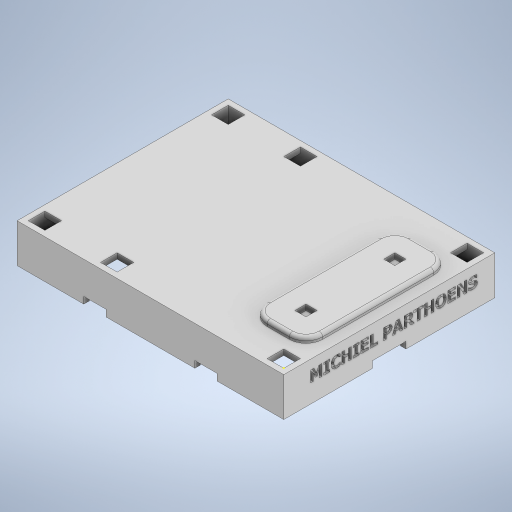
# Autodesk Inventor part: bovenkant
Saved by Autodesk Inventor 2023 (Build 270158000, 158)
## iProperties
Created: 2023-06-01
Part Number: bovenkant
Material: Generic
Document SubType Name: Modeling
Designer: Prestige
Density: 1 g/cm^3
Appearance: Default
Author: Prestige
Autodesk Inventor part; units mm, degrees
ref_plane "YZ Plane" through (0, 0, 0) normal (1, 0, 0) x (0, 1, 0)
ref_plane "XZ Plane" through (0, 0, 0) normal (0, 1, 0) x (-1, 0, 0)
ref_plane "XY Plane" through (0, 0, 0) normal (0, 0, 1) x (1, 0, 0)
sketch "Sketch1" plane through (0, 0, 0) normal (0, 1, 0) x (-1, 0, 0)
  line L0 (0, 0) -> (230, 0)
  line L1 (230, 0) -> (230, -180)
  line L2 (230, -180) -> (0, -180)
  line L3 (0, -180) -> (0, 0)
  line L4 (235, -185) -> (-5, -185)
  line L5 (-5, -185) -> (-5, 5)
  line L6 (-5, 5) -> (235, 5)
  line L7 (235, 5) -> (235, -185)
  line L8 (235, -75) -> (230, -75)
  line L9 (230, -75) -> (230, -105)
  line L10 (230, -105) -> (235, -105)
  line L11 (235, -105) -> (235, -75)
  line L12 (175, -180) -> (155, -180)
  line L13 (155, -180) -> (155, -185)
  line L14 (155, -185) -> (175, -185)
  line L15 (175, -185) -> (175, -180)
  line L16 (115, -180) -> (95, -180)
  line L17 (95, -185) -> (115, -185)
  line L18 (-5, -73.4747) -> (0, -73.4747)
  line L19 (0, -73.4747) -> (0, -111.2886)
  line L20 (0, -111.2886) -> (-5, -111.2886)
  line L21 (-5, -111.2886) -> (-5, -73.4747)
  line L22 (175, 0) -> (155, 0)
  line L23 (155, 0) -> (155, 5)
  line L24 (155, 5) -> (175, 5)
  line L25 (175, 5) -> (175, 0)
  line L26 (75, 0) -> (55, 0)
  line L27 (55, 0) -> (55, 5)
  line L28 (55, 5) -> (75, 5)
  line L29 (75, 5) -> (75, 0)
  line L30 (75, -180) -> (55, -180)
  line L31 (55, -180) -> (55, -185)
  line L32 (55, -185) -> (75, -185)
  line L33 (75, -185) -> (75, -180)
  point P0 (232.5, -75)
  point P1 (232.5, -105)
  point P2 (175, 2.5)
  point P3 (155, 2.5)
  point P4 (55, 2.5)
  point P5 (75, 2.5)
  point P6 (155, -182.5)
  point P7 (175, -182.5)
  point P8 (55, -182.5)
  point P9 (75, -182.5)
  point P10 (-5, -111.2886)
  point P11 (0, -73.4747)
  dimension "d0" = 180
  dimension "d1" = 230
  dimension "d2" = 5
  dimension "d3" = 5
  dimension "d4" = 5
  dimension "d5" = 5
  dimension "d6" = 30
  dimension "d7" = 75
  dimension "d8" = 75
  dimension "d9" = 20
  dimension "d10" = 20
  dimension "d12" = 20
  dimension "d14" = 80
  dimension "d15" = 55
  dimension "d16" = 55
  dimension "d17" = 20
  dimension "d18" = 80
  constraints: 68 end point, 17 parallel, 13 point on line, 11 midpoint, 9 horizontal, 8 perpendicular
  measures "d0" distance of L2.end L0.start
  measures "d1" distance of L0.start L0.end
  measures "d2" distance between parallel lines of L1 L7
  measures "d3" distance between parallel lines of L2 L4
  measures "d4" distance between parallel lines of L3 L5
  measures "d5" distance between parallel lines of L0 L6
  measures "d6" distance from line of point (232.5, -75) L10
  measures "d7" distance between parallel lines of L0 L8
  measures "d8" distance from line of L2 point (232.5, -105)
  measures "d9" distance of point (175, 2.5) point (155, 2.5)
  measures "d10" distance of point (55, 2.5) point (75, 2.5)
  measures "d12" distance of point (155, -182.5) point (175, -182.5)
  measures "d14" distance between parallel lines of L23 L29
  measures "d15" distance between parallel lines of L1 L25
  measures "d16" distance between parallel lines of L1 L15
  measures "d17" distance of point (55, -182.5) point (75, -182.5)
  measures "d18" distance from line of point (155, -182.5) L33
extrude "Extrusion1" add sketch "Sketch1" along normal blind 6 contours L3 L18 L5 L6 L27 L0 | L29 L6 L23 L0 | L3 L2 L31 L4 L5 L20 | L25 L6 L7 L8 L1 L0 | L2 L13 L4 L33 | L10 L7 L4 L15 L2 L1
sketch "Sketch2" plane through (0, 6, 0) normal (0, 1, 0) x (1, 0, 0)
  line L0 (0, 180) -> (0, 111.2886) projected
  line L1 (-175, 0) -> (-230, 0) projected
  line L2 (0, 180) -> (-230, 180)
  line L3 (-230, 180) -> (-230, 0)
  line L4 (-230, 0) -> (0, 0)
  line L5 (0, 0) -> (0, 180)
  line L6 (-235, 75) -> (-235, -5) projected
  line L7 (5, 111.2886) -> (5, 185) projected
  line L8 (-235, -5) -> (5, -5)
  line L9 (5, -5) -> (5, 185)
  line L10 (5, 185) -> (-235, 185)
  line L11 (-235, 185) -> (-235, -5)
  point P0 (0, 0)
  constraints: 16 end point, 4 parallel, 2 horizontal, 2 perpendicular
extrude "Extrusion2" add sketch "Sketch2" along normal blind 24
sketch "Sketch3" plane through (0, 30, 0) normal (0, 1, 0) x (1, 0, 0)
  line L0 (-235, -5) -> (5, -5) projected
  line L1 (5, 185) -> (-235, 185) projected
  line L2 (-235, -5) -> (5, -5)
  line L3 (5, -5) -> (5, 185)
  line L4 (5, 185) -> (-235, 185)
  line L5 (-235, 185) -> (-235, -5)
  point P0 (0, 0)
  constraints: 8 end point, 2 parallel, 1 horizontal, 1 perpendicular
extrude "Extrusion3" add sketch "Sketch3" along normal blind 5
sketch "Sketch4" plane through (0, 35, 0) normal (0, 1, 0) x (1, 0, 0)
  line L0 (-5, 25) -> (-55, 25)
  line L1 (-55, 25) -> (-55, 155)
  line L2 (-55, 155) -> (-5, 155)
  line L3 (-5, 155) -> (-5, 25)
  line L4 (5, 185) -> (-235, 185) projected
  line L5 (-235, -5) -> (5, -5) projected
  line L6 (5, -5) -> (5, 185) projected
  point P0 (0, 0)
  dimension "d25" = 130
  dimension "d26" = 30
  dimension "d27" = 30
  dimension "d28" = 10
  dimension "d29" = 50
  constraints: 8 end point, 2 parallel, 1 horizontal, 1 perpendicular
  measures "d25" distance of L0.end L1.end
  measures "d26" distance between parallel lines of L4 L2
  measures "d27" distance between parallel lines of L5 L0
  measures "d28" distance between parallel lines of L6 L3
  measures "d29" distance of L1.end L2.end
extrude "Extrusion4" add sketch "Sketch4" along normal blind 5
fillet "Fillet1" radius 15 4 edges at (-5, 37.5, -25) (-55, 37.5, -25) (-5, 37.5, -155) (-55, 37.5, -155)
fillet "Fillet2" radius 3 8 edges at (-9.3934, 40, -150.6066) (-30, 40, -155) (-50.6066, 40, -150.6066) (-55, 40, -90) (-50.6066, 40, -29.3934) (-30, 40, -25) (-9.3934, 40, -29.3934) (-5, 40, -90)
sketch "Sketch5" plane through (0, 40, 0) normal (0, 1, 0) x (1, 0, 0)
  line L0 (-25, 125) -> (-35, 125)
  line L1 (-35, 125) -> (-35, 135)
  line L2 (-35, 135) -> (-25, 135)
  line L3 (-25, 135) -> (-25, 125)
  line L4 (-20, 155) -> (-40, 155) projected
  line L5 (-55, 140) -> (-55, 40) projected
  line L6 (-35, 45) -> (-25, 45)
  line L7 (-25, 45) -> (-25, 55)
  line L8 (-25, 55) -> (-35, 55)
  line L9 (-35, 55) -> (-35, 45)
  line L10 (-40, 25) -> (-20, 25) projected
  point P0 (0, 0)
  point P1 (-30, 125)
  point P2 (-30, 155)
  point P3 (-30, 135)
  point P4 (-30, 45)
  point P5 (-35, 50)
  point P6 (-30, 25)
  dimension "d34" = 10
  dimension "d35" = 10
  dimension "d36" = 20
  dimension "d37" = 20
  dimension "d40" = 10
  dimension "d41" = 10
  dimension "d42" = 20
  dimension "d43" = 20
  constraints: 16 end point, 6 midpoint, 4 parallel, 2 horizontal, 2 perpendicular
  measures "d34" distance between parallel lines of L3 L1
  measures "d35" distance from line of point (-30, 125) L2
  measures "d36" distance of point (-30, 155) point (-30, 135)
  measures "d37" distance between parallel lines of L5 L1
  measures "d40" distance between parallel lines of L7 L9
  measures "d41" distance from line of point (-30, 45) L8
  measures "d42" distance from line of L5 point (-35, 50)
  measures "d43" distance of point (-30, 25) point (-30, 45)
extrude "Extrusion5" cut sketch "Sketch5" against normal blind 5
sketch "Sketch6" plane through (0, 35, 0) normal (0, 1, 0) x (1, 0, 0)
  line L0 (0, 0) -> (-55, 0) projected
  line L1 (0, 0) -> (-15, 0)
  line L2 (-15, 0) -> (-15, 15)
  line L3 (-15, 15) -> (0, 15)
  line L4 (0, 15) -> (0, 0)
  line L5 (5, -5) -> (5, 185) projected
  line L6 (0, 0) -> (-230, 0) projected
  line L7 (-230, 0) -> (-215, 0)
  line L8 (-215, 0) -> (-215, 15)
  line L9 (-215, 15) -> (-230, 15)
  line L10 (-230, 15) -> (-230, 0)
  line L11 (-230, 180) -> (-215, 180)
  line L12 (-215, 180) -> (-215, 165)
  line L13 (-215, 165) -> (-230, 165)
  line L14 (-230, 165) -> (-230, 180)
  line L15 (-165, 0) -> (-150, 0)
  line L16 (-150, 0) -> (-150, 15)
  line L17 (-150, 15) -> (-165, 15)
  line L18 (-165, 15) -> (-165, 0)
  line L19 (-165, 180) -> (-150, 180)
  line L20 (-150, 180) -> (-150, 165)
  line L21 (-150, 165) -> (-165, 165)
  line L22 (-165, 165) -> (-165, 180)
  line L23 (0, 180) -> (-15, 180)
  line L24 (-15, 180) -> (-15, 165)
  line L25 (-15, 165) -> (0, 165)
  line L26 (0, 165) -> (0, 180)
  point P0 (-222.5, 0)
  point P1 (-222.5, 15)
  dimension "d46" = 15
  dimension "d47" = 15
  dimension "d51" = 15
  dimension "d52" = 15
  dimension "d53" = 15
  dimension "d54" = 15
  dimension "d55" = 15
  dimension "d56" = 15
  dimension "d57" = 15
  dimension "d58" = 15
  dimension "d59" = 50
  dimension "d64" = 15
  dimension "d65" = 15
  constraints: 48 end point, 12 parallel, 6 horizontal, 6 perpendicular, 2 midpoint, 2 point on line
  measures "d46" distance of L1.end L2.end
  measures "d47" distance of L2.end L3.end
  measures "d51" distance of point (-222.5, 0) point (-222.5, 15)
  measures "d52" distance of L8.end L9.end
  measures "d53" distance of L11.end L12.end
  measures "d54" distance of L12.end L13.end
  measures "d55" distance of L17.end L15.start
  measures "d56" distance of L16.end L17.end
  measures "d57" distance of L20.end L21.end
  measures "d58" distance of L19.end L20.end
  measures "d59" distance between parallel lines of L12 L22
  measures "d64" distance of L24.end L25.end
  measures "d65" distance of L23.end L24.end
extrude "Extrusion6" cut sketch "Sketch6" against normal blind 5
sketch "Sketch7" plane through (5, 0, 5) normal (1, 0, 0) x (0, 0, -1)
  line L0 (110, 0) -> (110, 6) projected
  line L1 (110, 0) -> (120.7181, 0)
  line L2 (120.7181, 0) -> (120.7181, 6)
  line L3 (120.7181, 6) -> (110, 6)
  line L4 (110, 6) -> (110, 0)
  line L5 (80, 0) -> (80, 6) projected
  line L6 (80, 0) -> (68.1544, 0)
  line L7 (68.1544, 0) -> (68.1544, 6)
  line L8 (68.1544, 6) -> (80, 6)
  line L9 (80, 6) -> (80, 0)
  point P0 (5, 0)
  constraints: 16 end point, 4 parallel, 2 horizontal, 2 perpendicular
extrude "Extrusion7" add sketch "Sketch7" against normal blind 5
sketch "Sketch8" plane through (0, 35, 0) normal (0, 1, 0) x (1, 0, 0)
  point P0 (0, 0)
sketch "Sketch9" plane through (5, 0, -185) normal (1, 0, 0) x (0, 0, -1)
  line L0 (-166.856, 26.7371) -> (9.2467, 26.7371) construction
  line L1 (9.2467, 26.7371) -> (9.2467, 5.0092) construction
  line L2 (9.2467, 5.0092) -> (-166.856, 5.0092) construction
  line L3 (-166.856, 5.0092) -> (-166.856, 26.7371) construction
  line L4 (-155.608, 16.5264) -> (-158.104, 16.5264)
  line L5 (-158.104, 16.5264) -> (-158.104, 23.1553)
  line L6 (-158.104, 23.1553) -> (-159.9192, 18.8765)
  line L7 (-159.9192, 18.8765) -> (-161.6372, 18.8765)
  line L8 (-161.6372, 18.8765) -> (-163.4524, 23.1553)
  line L9 (-163.4524, 23.1553) -> (-163.4524, 16.5264)
  line L10 (-163.4524, 16.5264) -> (-165.8187, 16.5264)
  line L11 (-165.8187, 16.5264) -> (-165.8187, 26.5264)
  line L12 (-165.8187, 26.5264) -> (-162.9257, 26.5264)
  line L13 (-162.9257, 26.5264) -> (-160.7053, 21.5912)
  line L14 (-160.7053, 21.5912) -> (-158.501, 26.5264)
  line L15 (-158.501, 26.5264) -> (-155.608, 26.5264)
  line L16 (-155.608, 26.5264) -> (-155.608, 16.5264)
  line L17 (-148.5578, 16.5264) -> (-153.9386, 16.5264)
  line L18 (-153.9386, 16.5264) -> (-153.9386, 18.2687)
  line L19 (-153.9386, 18.2687) -> (-152.5043, 18.2687)
  line L20 (-152.5043, 18.2687) -> (-152.5043, 24.7841)
  line L21 (-152.5043, 24.7841) -> (-153.9386, 24.7841)
  line L22 (-153.9386, 24.7841) -> (-153.9386, 26.5264)
  line L23 (-153.9386, 26.5264) -> (-148.5578, 26.5264)
  line L24 (-148.5578, 26.5264) -> (-148.5578, 24.7841)
  line L25 (-148.5578, 24.7841) -> (-149.9921, 24.7841)
  line L26 (-149.9921, 24.7841) -> (-149.9921, 18.2687)
  line L27 (-149.9921, 18.2687) -> (-148.5578, 18.2687)
  line L28 (-148.5578, 18.2687) -> (-148.5578, 16.5264)
  spline S0 degree 2 poles (-142.5772, 16.3319) (-144.8301, 16.3319) (-147.4719, 19.0548) (-147.4719, 21.5183) knots 0 0 0 1 2 2 2
  spline S1 degree 2 poles (-147.4719, 21.5183) (-147.4719, 23.8927) (-144.8219, 26.7209) (-142.5691, 26.7209) knots 0 0 0 1 2 2 2
  spline S2 degree 2 poles (-142.5691, 26.7209) (-141.9775, 26.7209) (-141.0213, 26.5831) (-140.5837, 26.4697) knots 0 0 0 1 2 2 2
  spline S3 degree 2 poles (-140.5837, 26.4697) (-140.2433, 26.3643) (-139.4411, 26.0159) (-139.1899, 25.8862) knots 0 0 0 1 2 2 2
  line L29 (-139.1899, 25.8862) -> (-139.1899, 23.5037)
  line L30 (-139.1899, 23.5037) -> (-139.4411, 23.5037)
  spline S4 degree 2 poles (-139.4411, 23.5037) (-139.6275, 23.6658) (-140.1785, 24.1196) (-140.527, 24.3303) knots 0 0 0 1 2 2 2
  spline S5 degree 2 poles (-140.527, 24.3303) (-140.8754, 24.5491) (-141.7101, 24.8489) (-142.172, 24.8489) knots 0 0 0 1 2 2 2
  spline S6 degree 2 poles (-142.172, 24.8489) (-142.715, 24.8489) (-143.6145, 24.5086) (-144.0278, 24.0791) knots 0 0 0 1 2 2 2
  spline S7 degree 2 poles (-144.0278, 24.0791) (-144.4006, 23.6982) (-144.8787, 22.3935) (-144.8787, 21.5102) knots 0 0 0 1 2 2 2
  spline S8 degree 2 poles (-144.8787, 21.5102) (-144.8787, 20.5783) (-144.3843, 19.306) (-143.9792, 18.917) knots 0 0 0 1 2 2 2
  spline S9 degree 2 poles (-143.9792, 18.917) (-143.5902, 18.5361) (-142.6339, 18.2039) (-142.1558, 18.2039) knots 0 0 0 1 2 2 2
  spline S10 degree 2 poles (-142.1558, 18.2039) (-141.6615, 18.2039) (-140.762, 18.5361) (-140.454, 18.7387) knots 0 0 0 1 2 2 2
  spline S11 degree 2 poles (-140.454, 18.7387) (-140.1137, 18.9413) (-139.6031, 19.3708) (-139.4168, 19.541) knots 0 0 0 1 2 2 2
  line L31 (-139.4168, 19.541) -> (-139.1899, 19.541)
  line L32 (-139.1899, 19.541) -> (-139.1899, 17.1909)
  spline S12 degree 2 poles (-139.1899, 17.1909) (-139.4654, 17.0612) (-140.1866, 16.7371) (-140.5756, 16.6236) knots 0 0 0 1 2 2 2
  spline S13 degree 2 poles (-140.5756, 16.6236) (-141.0456, 16.4778) (-141.8641, 16.3319) (-142.5772, 16.3319) knots 0 0 0 1 2 2 2
  line L33 (-129.2709, 16.5264) -> (-131.7831, 16.5264)
  line L34 (-131.7831, 16.5264) -> (-131.7831, 20.9591)
  line L35 (-131.7831, 20.9591) -> (-135.1947, 20.9591)
  line L36 (-135.1947, 20.9591) -> (-135.1947, 16.5264)
  line L37 (-135.1947, 16.5264) -> (-137.7069, 16.5264)
  line L38 (-137.7069, 16.5264) -> (-137.7069, 26.5264)
  line L39 (-137.7069, 26.5264) -> (-135.1947, 26.5264)
  line L40 (-135.1947, 26.5264) -> (-135.1947, 22.8635)
  line L41 (-135.1947, 22.8635) -> (-131.7831, 22.8635)
  line L42 (-131.7831, 22.8635) -> (-131.7831, 26.5264)
  line L43 (-131.7831, 26.5264) -> (-129.2709, 26.5264)
  line L44 (-129.2709, 26.5264) -> (-129.2709, 16.5264)
  line L45 (-122.2207, 16.5264) -> (-127.6015, 16.5264)
  line L46 (-127.6015, 16.5264) -> (-127.6015, 18.2687)
  line L47 (-127.6015, 18.2687) -> (-126.1672, 18.2687)
  line L48 (-126.1672, 18.2687) -> (-126.1672, 24.7841)
  line L49 (-126.1672, 24.7841) -> (-127.6015, 24.7841)
  line L50 (-127.6015, 24.7841) -> (-127.6015, 26.5264)
  line L51 (-127.6015, 26.5264) -> (-122.2207, 26.5264)
  line L52 (-122.2207, 26.5264) -> (-122.2207, 24.7841)
  line L53 (-122.2207, 24.7841) -> (-123.655, 24.7841)
  line L54 (-123.655, 24.7841) -> (-123.655, 18.2687)
  line L55 (-123.655, 18.2687) -> (-122.2207, 18.2687)
  line L56 (-122.2207, 18.2687) -> (-122.2207, 16.5264)
  line L57 (-120.5513, 16.5264) -> (-120.5513, 26.5264)
  line L58 (-120.5513, 26.5264) -> (-113.7928, 26.5264)
  line L59 (-113.7928, 26.5264) -> (-113.7928, 24.622)
  line L60 (-113.7928, 24.622) -> (-118.0553, 24.622)
  line L61 (-118.0553, 24.622) -> (-118.0553, 22.8635)
  line L62 (-118.0553, 22.8635) -> (-114.125, 22.8635)
  line L63 (-114.125, 22.8635) -> (-114.125, 20.9591)
  line L64 (-114.125, 20.9591) -> (-118.0553, 20.9591)
  line L65 (-118.0553, 20.9591) -> (-118.0553, 18.4308)
  line L66 (-118.0553, 18.4308) -> (-113.7928, 18.4308)
  line L67 (-113.7928, 18.4308) -> (-113.7928, 16.5264)
  line L68 (-113.7928, 16.5264) -> (-120.5513, 16.5264)
  line L69 (-105.4216, 16.5264) -> (-112.091, 16.5264)
  line L70 (-112.091, 16.5264) -> (-112.091, 26.5264)
  line L71 (-112.091, 26.5264) -> (-109.5788, 26.5264)
  line L72 (-109.5788, 26.5264) -> (-109.5788, 18.4308)
  line L73 (-109.5788, 18.4308) -> (-105.4216, 18.4308)
  line L74 (-105.4216, 18.4308) -> (-105.4216, 16.5264)
  spline S14 degree 2 poles (-92.5043, 23.3741) (-92.5043, 22.6771) (-92.95, 21.4129) (-93.3633, 20.9916) knots 0 0 0 1 2 2 2
  spline S15 degree 2 poles (-93.3633, 20.9916) (-93.6145, 20.7241) (-94.2304, 20.2865) (-94.595, 20.1326) knots 0 0 0 1 2 2 2
  spline S16 degree 2 poles (-94.595, 20.1326) (-94.9678, 19.9786) (-95.8349, 19.8003) (-96.3698, 19.8003) knots 0 0 0 1 2 2 2
  line L75 (-96.3698, 19.8003) -> (-97.6826, 19.8003)
  line L76 (-97.6826, 19.8003) -> (-97.6826, 16.5264)
  line L77 (-97.6826, 16.5264) -> (-100.1947, 16.5264)
  line L78 (-100.1947, 16.5264) -> (-100.1947, 26.5264)
  line L79 (-100.1947, 26.5264) -> (-96.313, 26.5264)
  spline S17 degree 2 poles (-96.313, 26.5264) (-95.454, 26.5264) (-94.198, 26.2104) (-93.6874, 25.87) knots 0 0 0 1 2 2 2
  spline S18 degree 2 poles (-93.6874, 25.87) (-93.1202, 25.4891) (-92.5043, 24.2412) (-92.5043, 23.3741) knots 0 0 0 1 2 2 2
  spline S19 degree 2 poles (-95.0813, 23.3092) (-95.0813, 23.7387) (-95.4865, 24.3465) (-95.762, 24.46) knots 0 0 0 1 2 2 2
  spline S20 degree 2 poles (-95.762, 24.46) (-96.1185, 24.6139) (-96.7668, 24.6625) (-97.326, 24.6625) knots 0 0 0 1 2 2 2
  line L80 (-97.326, 24.6625) -> (-97.6826, 24.6625)
  line L81 (-97.6826, 24.6625) -> (-97.6826, 21.6642)
  line L82 (-97.6826, 21.6642) -> (-97.5043, 21.6642)
  spline S21 degree 2 poles (-97.5043, 21.6642) (-97.1558, 21.6642) (-96.5237, 21.6804) (-96.2887, 21.7209) knots 0 0 0 1 2 2 2
  spline S22 degree 2 poles (-96.2887, 21.7209) (-96.0861, 21.7533) (-95.6404, 21.9478) (-95.5189, 22.0694) knots 0 0 0 1 2 2 2
  spline S23 degree 2 poles (-95.5189, 22.0694) (-95.2595, 22.3125) (-95.0813, 22.8554) (-95.0813, 23.3092) knots 0 0 0 1 2 2 2
  line L83 (-92.2369, 16.5264) -> (-88.8576, 26.5264)
  line L84 (-88.8576, 26.5264) -> (-86.1185, 26.5264)
  line L85 (-86.1185, 26.5264) -> (-82.7393, 16.5264)
  line L86 (-82.7393, 16.5264) -> (-85.3244, 16.5264)
  line L87 (-85.3244, 16.5264) -> (-85.9484, 18.5685)
  line L88 (-85.9484, 18.5685) -> (-89.0926, 18.5685)
  line L89 (-89.0926, 18.5685) -> (-89.7247, 16.5264)
  line L90 (-89.7247, 16.5264) -> (-92.2369, 16.5264)
  line L91 (-86.4994, 20.3838) -> (-87.5205, 23.6901)
  line L92 (-87.5205, 23.6901) -> (-88.5497, 20.3838)
  line L93 (-88.5497, 20.3838) -> (-86.4994, 20.3838)
  line L94 (-72.5043, 16.5264) -> (-75.5594, 16.5264)
  line L95 (-75.5594, 16.5264) -> (-78.339, 20.1974)
  line L96 (-78.339, 20.1974) -> (-79.2466, 20.1974)
  line L97 (-79.2466, 20.1974) -> (-79.2466, 16.5264)
  line L98 (-79.2466, 16.5264) -> (-81.7425, 16.5264)
  line L99 (-81.7425, 16.5264) -> (-81.7425, 26.5264)
  line L100 (-81.7425, 26.5264) -> (-77.7231, 26.5264)
  spline S24 degree 2 poles (-77.7231, 26.5264) (-76.8884, 26.5264) (-75.6566, 26.3157) (-75.1299, 25.9916) knots 0 0 0 1 2 2 2
  spline S25 degree 2 poles (-75.1299, 25.9916) (-74.595, 25.6512) (-73.963, 24.5896) (-73.963, 23.7792) knots 0 0 0 1 2 2 2
  spline S26 degree 2 poles (-73.963, 23.7792) (-73.963, 22.6366) (-75.0002, 21.2023) (-75.8673, 20.7809) knots 0 0 0 1 2 2 2
  line L101 (-75.8673, 20.7809) -> (-72.5043, 16.5264)
  spline S27 degree 2 poles (-76.5399, 23.4632) (-76.5399, 23.8441) (-76.8317, 24.387) (-77.1639, 24.5329) knots 0 0 0 1 2 2 2
  spline S28 degree 2 poles (-77.1639, 24.5329) (-77.3989, 24.6301) (-77.9743, 24.6869) (-78.4038, 24.6869) knots 0 0 0 1 2 2 2
  line L102 (-78.4038, 24.6869) -> (-79.2466, 24.6869)
  line L103 (-79.2466, 24.6869) -> (-79.2466, 21.9964)
  line L104 (-79.2466, 21.9964) -> (-78.5254, 21.9964)
  spline S29 degree 2 poles (-78.5254, 21.9964) (-78.0067, 21.9964) (-77.2693, 22.1261) (-77.0181, 22.3287) knots 0 0 0 1 2 2 2
  spline S30 degree 2 poles (-77.0181, 22.3287) (-76.7749, 22.5232) (-76.5399, 23.0418) (-76.5399, 23.4632) knots 0 0 0 1 2 2 2
  line L105 (-69.8382, 16.5264) -> (-69.8382, 24.622)
  line L106 (-69.8382, 24.622) -> (-72.796, 24.622)
  line L107 (-72.796, 24.622) -> (-72.796, 26.5264)
  line L108 (-72.796, 26.5264) -> (-64.3681, 26.5264)
  line L109 (-64.3681, 26.5264) -> (-64.3681, 24.622)
  line L110 (-64.3681, 24.622) -> (-67.326, 24.622)
  line L111 (-67.326, 24.622) -> (-67.326, 16.5264)
  line L112 (-67.326, 16.5264) -> (-69.8382, 16.5264)
  line L113 (-54.903, 16.5264) -> (-57.4151, 16.5264)
  line L114 (-57.4151, 16.5264) -> (-57.4151, 20.9591)
  line L115 (-57.4151, 20.9591) -> (-60.8268, 20.9591)
  line L116 (-60.8268, 20.9591) -> (-60.8268, 16.5264)
  line L117 (-60.8268, 16.5264) -> (-63.339, 16.5264)
  line L118 (-63.339, 16.5264) -> (-63.339, 26.5264)
  line L119 (-63.339, 26.5264) -> (-60.8268, 26.5264)
  line L120 (-60.8268, 26.5264) -> (-60.8268, 22.8635)
  line L121 (-60.8268, 22.8635) -> (-57.4151, 22.8635)
  line L122 (-57.4151, 22.8635) -> (-57.4151, 26.5264)
  line L123 (-57.4151, 26.5264) -> (-54.903, 26.5264)
  line L124 (-54.903, 26.5264) -> (-54.903, 16.5264)
  spline S31 degree 2 poles (-43.7279, 21.5264) (-43.7279, 19.0953) (-46.3211, 16.3157) (-48.574, 16.3157) knots 0 0 0 1 2 2 2
  spline S32 degree 2 poles (-48.574, 16.3157) (-50.8349, 16.3157) (-53.4119, 19.1277) (-53.4119, 21.5264) knots 0 0 0 1 2 2 2
  spline S33 degree 2 poles (-53.4119, 21.5264) (-53.4119, 23.9332) (-50.8349, 26.7371) (-48.574, 26.7371) knots 0 0 0 1 2 2 2
  spline S34 degree 2 poles (-48.574, 26.7371) (-46.3211, 26.7371) (-43.7279, 23.9494) (-43.7279, 21.5264) knots 0 0 0 1 2 2 2
  spline S35 degree 2 poles (-46.3211, 21.5264) (-46.3211, 22.4259) (-46.6858, 23.682) (-47.0019, 24.0791) knots 0 0 0 1 2 2 2
  spline S36 degree 2 poles (-47.0019, 24.0791) (-47.3179, 24.4924) (-48.1283, 24.8489) (-48.5659, 24.8489) knots 0 0 0 1 2 2 2
  spline S37 degree 2 poles (-48.5659, 24.8489) (-49.0278, 24.8489) (-49.7814, 24.5167) (-50.1299, 24.0953) knots 0 0 0 1 2 2 2
  spline S38 degree 2 poles (-50.1299, 24.0953) (-50.4378, 23.7063) (-50.8187, 22.4178) (-50.8187, 21.5264) knots 0 0 0 1 2 2 2
  spline S39 degree 2 poles (-50.8187, 21.5264) (-50.8187, 20.6026) (-50.454, 19.387) (-50.138, 18.9737) knots 0 0 0 1 2 2 2
  spline S40 degree 2 poles (-50.138, 18.9737) (-49.8219, 18.5604) (-49.0035, 18.2039) (-48.5659, 18.2039) knots 0 0 0 1 2 2 2
  spline S41 degree 2 poles (-48.5659, 18.2039) (-48.1202, 18.2039) (-47.2936, 18.5847) (-46.9937, 18.9899) knots 0 0 0 1 2 2 2
  spline S42 degree 2 poles (-46.9937, 18.9899) (-46.6696, 19.4275) (-46.3211, 20.5864) (-46.3211, 21.5264) knots 0 0 0 1 2 2 2
  line L125 (-42.2369, 16.5264) -> (-42.2369, 26.5264)
  line L126 (-42.2369, 26.5264) -> (-35.4784, 26.5264)
  line L127 (-35.4784, 26.5264) -> (-35.4784, 24.622)
  line L128 (-35.4784, 24.622) -> (-39.7409, 24.622)
  line L129 (-39.7409, 24.622) -> (-39.7409, 22.8635)
  line L130 (-39.7409, 22.8635) -> (-35.8106, 22.8635)
  line L131 (-35.8106, 22.8635) -> (-35.8106, 20.9591)
  line L132 (-35.8106, 20.9591) -> (-39.7409, 20.9591)
  line L133 (-39.7409, 20.9591) -> (-39.7409, 18.4308)
  line L134 (-39.7409, 18.4308) -> (-35.4784, 18.4308)
  line L135 (-35.4784, 18.4308) -> (-35.4784, 16.5264)
  line L136 (-35.4784, 16.5264) -> (-42.2369, 16.5264)
  line L137 (-25.2109, 16.5264) -> (-27.6258, 16.5264)
  line L138 (-27.6258, 16.5264) -> (-31.4832, 23.4956)
  line L139 (-31.4832, 23.4956) -> (-31.4832, 16.5264)
  line L140 (-31.4832, 16.5264) -> (-33.7766, 16.5264)
  line L141 (-33.7766, 16.5264) -> (-33.7766, 26.5264)
  line L142 (-33.7766, 26.5264) -> (-30.6972, 26.5264)
  line L143 (-30.6972, 26.5264) -> (-27.5043, 20.7971)
  line L144 (-27.5043, 20.7971) -> (-27.5043, 26.5264)
  line L145 (-27.5043, 26.5264) -> (-25.2109, 26.5264)
  line L146 (-25.2109, 26.5264) -> (-25.2109, 16.5264)
  spline S43 degree 2 poles (-20.0894, 16.3481) (-21.2401, 16.3481) (-22.9743, 16.7938) (-23.7198, 17.118) knots 0 0 0 1 2 2 2
  line L147 (-23.7198, 17.118) -> (-23.7198, 19.5005)
  line L148 (-23.7198, 19.5005) -> (-23.4929, 19.5005)
  spline S44 degree 2 poles (-23.4929, 19.5005) (-22.7393, 18.8603) (-20.9322, 18.1715) (-20.0813, 18.1715) knots 0 0 0 1 2 2 2
  spline S45 degree 2 poles (-20.0813, 18.1715) (-19.8625, 18.1715) (-19.1574, 18.2687) (-18.9467, 18.3659) knots 0 0 0 1 2 2 2
  spline S46 degree 2 poles (-18.9467, 18.3659) (-18.6874, 18.4794) (-18.3228, 18.8927) (-18.3228, 19.2249) knots 0 0 0 1 2 2 2
  spline S47 degree 2 poles (-18.3228, 19.2249) (-18.3228, 19.6058) (-18.9143, 20.0758) (-19.3195, 20.1812) knots 0 0 0 1 2 2 2
  spline S48 degree 2 poles (-19.3195, 20.1812) (-19.8301, 20.3189) (-20.9889, 20.554) (-21.4994, 20.7322) knots 0 0 0 1 2 2 2
  spline S49 degree 2 poles (-21.4994, 20.7322) (-22.6583, 21.1374) (-23.6631, 22.5232) (-23.6631, 23.5604) knots 0 0 0 1 2 2 2
  spline S50 degree 2 poles (-23.6631, 23.5604) (-23.6631, 24.9624) (-21.2887, 26.7047) (-19.5059, 26.7047) knots 0 0 0 1 2 2 2
  spline S51 degree 2 poles (-19.5059, 26.7047) (-18.6145, 26.7047) (-16.8479, 26.34) (-16.151, 26.0321) knots 0 0 0 1 2 2 2
  line L149 (-16.151, 26.0321) -> (-16.151, 23.7468)
  line L150 (-16.151, 23.7468) -> (-16.3698, 23.7468)
  spline S52 degree 2 poles (-16.3698, 23.7468) (-16.9289, 24.2249) (-18.5335, 24.8813) (-19.3762, 24.8813) knots 0 0 0 1 2 2 2
  spline S53 degree 2 poles (-19.3762, 24.8813) (-19.7085, 24.8813) (-20.2271, 24.7841) (-20.5189, 24.6544) knots 0 0 0 1 2 2 2
  spline S54 degree 2 poles (-20.5189, 24.6544) (-20.7539, 24.5491) (-21.0942, 24.1277) (-21.0942, 23.8684) knots 0 0 0 1 2 2 2
  spline S55 degree 2 poles (-21.0942, 23.8684) (-21.0942, 23.4794) (-20.5513, 23.0337) (-19.7733, 22.8554) knots 0 0 0 1 2 2 2
  spline S56 degree 2 poles (-19.7733, 22.8554) (-19.2709, 22.742) (-18.339, 22.5232) (-17.8041, 22.3368) knots 0 0 0 1 2 2 2
  spline S57 degree 2 poles (-17.8041, 22.3368) (-16.7668, 21.9559) (-15.7539, 20.6917) (-15.7539, 19.6544) knots 0 0 0 1 2 2 2
  spline S58 degree 2 poles (-15.7539, 19.6544) (-15.7539, 18.1634) (-18.0959, 16.3481) (-20.0894, 16.3481) knots 0 0 0 1 2 2 2
  point P0 (-185, 0)
  constraints: 2 other
extrude "Extrusion8" cut sketch "Sketch9" against normal blind 2.5
body "Solid1"
